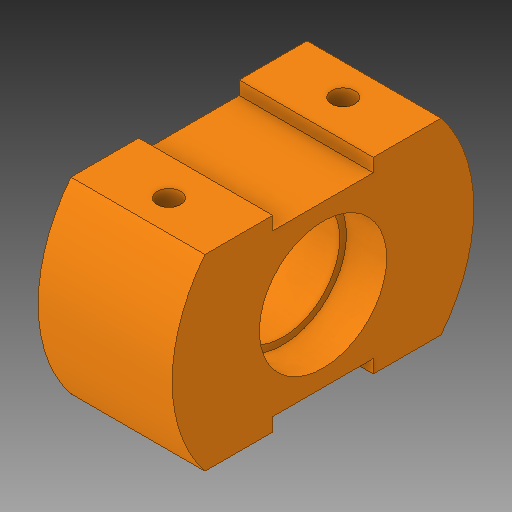
# Autodesk Inventor part: 04-04-Кулак
Saved by Autodesk Inventor 2018 (Build 220112000, 112)
## iProperties
Part Number: 04-04-Кулак
Material: Типовые
Document SubType Name: Modeling
Designer: sbnnl
Density: 1 g/cm^3
Appearance: Оранжевый
Author: sbnnl
Autodesk Inventor part; units mm, degrees
ref_plane "YZ Plane" through (0, 0, 0) normal (1, 0, 0) x (0, 1, 0)
ref_plane "XZ Plane" through (0, 0, 0) normal (0, 1, 0) x (-1, 0, 0)
ref_plane "XY Plane" through (0, 0, 0) normal (0, 0, 1) x (1, 0, 0)
sketch "Эскиз1" plane through (0, 0, 0) normal (1, 0, 0) x (0, 1, 0)
  circle A0 centre (0, 0) radius 8.5
  circle A1 centre (0, 0) radius 22.5
  dimension "d0" = 17
  dimension "d1" = 45
  constraints: 2 centre point, 2 coincident
  measures "d0" diameter of A0
  measures "d1" diameter of A1
extrude "Выдавливание1" add sketch "Эскиз1" along normal blind 20
sketch "Эскиз2" plane through (20, 0, 0) normal (1, 0, 0) x (0, 0, -1)
  circle A0 centre (0, 0) radius 9.5
  dimension "d4" = 19
  constraints: 1 centre point, 1 coincident
  measures "d4" diameter of A0
extrude "Выдавливание2" cut sketch "Эскиз2" against normal blind 6
sketch "Эскиз3" plane through (0, 0, 0) normal (-1, 0, 0) x (0, 0, 1)
  circle A0 centre (0, 0) radius 9.5
  dimension "d7" = 19
  constraints: 1 centre point, 1 coincident
  measures "d7" diameter of A0
extrude "Выдавливание3" cut sketch "Эскиз3" against normal blind 6
sketch "Эскиз4" plane through (0, 0, 0) normal (-1, 0, 0) x (0, 0, 1)
  line L0 (0, 0) -> (-20.5063, 0) construction
  line L1 (-25, -34) -> (25, -34)
  line L2 (25, -34) -> (25, -14)
  line L3 (25, -14) -> (-25, -14)
  line L4 (-25, -14) -> (-25, -34)
  line L5 (0, 0) -> (0, -5.1582) construction
  line L6 (-25, 34) -> (25, 34)
  line L7 (25, 34) -> (25, 14)
  line L8 (25, 14) -> (-25, 14)
  line L9 (-25, 14) -> (-25, 34)
  line L10 (7.5, -14) -> (-7.5, -14)
  line L11 (-7.5, -14) -> (-7.5, -12)
  line L12 (-7.5, -12) -> (7.5, -12)
  line L13 (7.5, -12) -> (7.5, -14)
  line L14 (7.5, 14) -> (-7.5, 14)
  line L15 (-7.5, 14) -> (-7.5, 12)
  line L16 (-7.5, 12) -> (7.5, 12)
  line L17 (7.5, 12) -> (7.5, 14)
  dimension "d10" = 20
  dimension "d11" = 50
  dimension "d12" = 14
  dimension "d18" = 2
  dimension "d19" = 15
  constraints: 36 end point, 8 symmetric about line, 4 parallel, 3 horizontal, 2 perpendicular, 1 point on line, 1 vertical, 2 other
  measures "d10" distance of L3.end L1.start
  measures "d11" distance between parallel lines of L2 L4
  measures "d12" distance between parallel lines of L3 L0
  measures "d18" distance of L10.end L11.end
  measures "d19" distance of L11.end L12.end
extrude "Выдавливание4" cut sketch "Эскиз4" against normal blind 50
sketch "Эскиз5" plane through (0, -14, -17.6139) normal (0, -1, 0) x (1, 0, 0)
  line L0 (0, 25.1139) -> (20, 25.1139) projected
  line L1 (10, 25.1139) -> (10, 12.2228) construction
  circle A0 centre (10, 30.6139) radius 1.75
  line L2 (0, 17.6139) -> (23.1932, 17.6139) construction
  circle A1 centre (10, 4.6139) radius 1.75
  dimension "d20" = 3.5
  dimension "d21" = 13
  constraints: 4 end point, 2 centre point, 1 horizontal, 1 midpoint, 1 point on line, 1 symmetric about line, 1 vertical, 1 other
  measures "d20" diameter of A0
  measures "d21" vertical distance of L2.start A0.centre
extrude "Выдавливание5" cut sketch "Эскиз5" against normal through all
